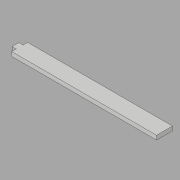
# Autodesk Inventor part: g_arm 4
Saved by Autodesk Inventor 2019 (Build 230136000, 136)
## iProperties
Created: 2021-11-01
Part Number: g_arm 4
Material: Generic
Document SubType Name: Modeling
Designer: Mohamed
Density: 1 g/cm^3
Appearance: Default
Author: Mohamed
Autodesk Inventor part; units mm, degrees
ref_plane "YZ Plane" through (0, 0, 0) normal (1, 0, 0) x (0, 1, 0)
ref_plane "XZ Plane" through (0, 0, 0) normal (0, 1, 0) x (-1, 0, 0)
ref_plane "XY Plane" through (0, 0, 0) normal (0, 0, 1) x (1, 0, 0)
sketch "Sketch1" plane through (0, 0, 0) normal (0, 1, 0) x (-1, 0, 0)
  line L0 (0, 0) -> (209, 0)
  line L1 (209, -23) -> (0, -23)
  line L2 (0, -23) -> (0, 0)
  line L3 (209, -6.5) -> (215, -6.5)
  line L4 (215, -6.5) -> (215, -16.5)
  line L5 (215, -16.5) -> (209, -16.5)
  line L6 (209, 0) -> (209, -6.5)
  line L7 (209, -16.5) -> (209, -23)
  dimension "d0" = 209
  dimension "d1" = 23
  dimension "d3" = 6
  dimension "d4" = 10
  constraints: 16 end point, 4 parallel, 3 perpendicular, 2 horizontal
  measures "d0" distance of L1.start L1.end
  measures "d1" distance of L0.end L1.start
  measures "d3" distance of L4.end L5.end
  measures "d4" distance of L3.end L4.end
extrude "Extrusion1" add sketch "Sketch1" along normal blind 6
body "Solid1"
